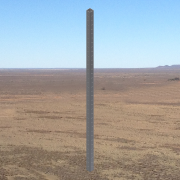
# Autodesk Inventor part: frame_uni_vert
Saved by Autodesk Inventor 2014 SP1 (Build 180222100, 222)
## iProperties
Created: 2014-05-23
Part Number: frame_uni_vert
Material: Steel, Mild
Document SubType Name: Modeling
Designer: Dave
Mass: 1021.47 g
Surface Area: 1671.74 cm^2
Volume: 129.958 cm^3
Density: 7.86 g/cm^3
Appearance: Steel
Author: Dave
Autodesk Inventor part; units mm, degrees
ref_plane "YZ Plane" through (0, 0, 0) normal (1, 0, 0) x (0, 1, 0)
ref_plane "XZ Plane" through (0, 0, 0) normal (0, 1, 0) x (-1, 0, 0)
ref_plane "XY Plane" through (0, 0, 0) normal (0, 0, 1) x (1, 0, 0)
sketch "Sketch1" plane through (0, 0, 0) normal (0, 1, 0) x (-1, 0, 0)
  line L0 (3.175, 0) -> (22.225, 0)
  line L1 (25.4, 3.175) -> (25.4, 22.225)
  line L2 (22.225, 25.4) -> (3.175, 25.4)
  line L3 (0, 22.225) -> (0, 3.175)
  arc A0 (25.4, 22.225) -> (22.225, 25.4) centre (22.225, 22.225) ccw
  arc A1 (22.225, 0) -> (25.4, 3.175) centre (22.225, 3.175) ccw
  arc A2 (0, 3.175) -> (3.175, 0) centre (3.175, 3.175) ccw
  arc A3 (3.175, 25.4) -> (0, 22.225) centre (3.175, 22.225) ccw
  line L4 (3.175, 23.8426) -> (22.225, 23.8426)
  arc A4 (23.8426, 22.225) -> (22.225, 23.8426) centre (22.225, 22.225) ccw
  line L5 (23.8426, 22.225) -> (23.8426, 3.175)
  arc A5 (22.225, 1.5574) -> (23.8426, 3.175) centre (22.225, 3.175) ccw
  line L6 (22.225, 1.5574) -> (3.175, 1.5574)
  arc A6 (1.5574, 3.175) -> (3.175, 1.5574) centre (3.175, 3.175) ccw
  line L7 (1.5574, 3.175) -> (1.5574, 22.225)
  arc A7 (3.175, 23.8426) -> (1.5574, 22.225) centre (3.175, 22.225) ccw
  point P0 (0, 0)
  point P1 (25.4, 25.4)
  point P2 (25.4, 0)
  point P3 (0, 25.4)
  dimension "d0" = 25.4
  dimension "d1" = 25.4
  dimension "d2" = 3.175
  constraints: 16 end point, 16 point on circle, 8 centre point, 8 point on line, 8 tangent, 4 parallel, 3 equal radius, 2 perpendicular, 1 horizontal, 7 other
  measures "d0" distance of point (0, 25.4) point (25.4, 25.4)
  measures "d1" distance of point (25.4, 25.4) point (25.4, 0)
  measures "d2" radius of A0
extrude "Extrusion1" add sketch "Sketch1" along normal blind 914.4
sketch "Sketch2" plane through (-22.225, 0, 25.4) normal (0, 0, 1) x (1, 0, 0)
  line L0 (19.05, 0) -> (0, 0) projected
  circle A0 centre (9.525, 25.4) radius 3.175
  point P0 (22.225, 0)
  dimension "d5" = 6.35
  dimension "d6" = 25.4
  constraints: 1 centre point
  measures "d5" diameter of A0
  measures "d6" distance from line of L0 A0.centre
hole "Hole1" at (-12.7, 25.4, 25.4) direction (0, 0, -1) diameter 6.35 end through all
pattern_linear "Rectangular Pattern1" count 35 spacing 25.4 along (0, 1, 0) of "Hole1"
sketch "Sketch3" plane through (0, 0, 22.225) normal (1, 0, 0) x (0, 0, -1)
  line L0 (19.05, 0) -> (0, 0) projected
  circle A0 centre (9.525, 25.4) radius 1.519
  point P0 (22.225, 0)
  dimension "d17" = 25.4
  constraints: 1 centre point
  measures "d17" distance from line of L0 A0.centre
hole "Hole2" at (0, 25.4, 12.7) direction (-1, 0, 0) diameter 6.35 end through all
pattern_linear "Rectangular Pattern2" count 35 spacing 25.4 along (0, 1, 0) of "Hole2"
body "Solid1"
